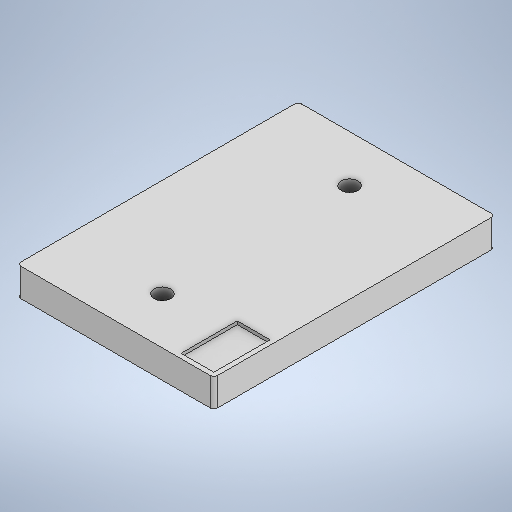
# Autodesk Inventor part: Podstawa
Saved by Autodesk Inventor 2025 (Build 290162000, 162)
## iProperties
Created: 2024-04-05
Part Number: Podstawa
Material: Generic
Document SubType Name: Modeling
Designer: Wojtek
Density: 1 g/cm^3
Appearance: Default
Author: Wojtek
Autodesk Inventor part; units mm, degrees
ref_plane "YZ Plane" through (0, 0, 0) normal (1, 0, 0) x (0, 1, 0)
ref_plane "XZ Plane" through (0, 0, 0) normal (0, 1, 0) x (-1, 0, 0)
ref_plane "XY Plane" through (0, 0, 0) normal (0, 0, 1) x (1, 0, 0)
sketch "Sketch1" plane through (0, 0, 0) normal (0, 1, 0) x (-1, 0, 0)
  line L0 (105, -150) -> (-105, -150)
  line L1 (-105, -150) -> (-105, 150)
  line L2 (-105, 150) -> (105, 150)
  line L3 (105, 150) -> (105, -150)
  line L4 (105, -150) -> (-105, 150) construction
  line L5 (-105, -150) -> (105, 150) construction
  point P0 (0, 0)
  dimension "d0" = 210
  dimension "d1" = 300
  constraints: 12 end point, 2 midpoint, 2 parallel, 1 horizontal, 1 perpendicular
  measures "d0" distance of L1.end L2.end
  measures "d1" distance of L0.end L1.end
extrude "Extrusion1" add sketch "Sketch1" along normal blind 30
sketch "Sketch2" plane through (0, 30, 0) normal (0, 1, 0) x (1, 0, 0)
  circle A0 centre (0, 100) radius 9
  circle A1 centre (0, -100) radius 9
  point P0 (0, 0)
  dimension "d4" = 18
  dimension "d5" = 18
  dimension "d6" = 100
  dimension "d7" = 100
  constraints: 2 centre point, 2 vertical alignment
  measures "d4" diameter of A0
  measures "d5" diameter of A1
  measures "d6" distance of point (0, 0) A0.centre
  measures "d7" distance of point (0, 0) A1.centre
hole "Hole1" at (0, 30, -100) at (0, 30, 100) direction (0, -1, 0) diameter 0.1 end through all counterbore diameter 18 counterbore depth 24
sketch "Sketch3" plane through (0, 30, 0) normal (0, 1, 0) x (1, 0, 0)
  line L0 (65, -145) -> (100, -145)
  line L1 (100, -145) -> (100, -85)
  line L2 (100, -85) -> (65, -85)
  line L3 (65, -85) -> (65, -145)
  line L4 (-105, -150) -> (105, -150) projected
  line L5 (105, -150) -> (105, 150) projected
  point P0 (0, 0)
  dimension "d15" = 35
  dimension "d16" = 60
  dimension "d17" = 5
  dimension "d19" = 5
  constraints: 8 end point, 2 parallel, 1 horizontal, 1 perpendicular
  measures "d15" distance of L2.end L1.end
  measures "d16" distance of L1.end L0.end
  measures "d17" distance between parallel lines of L4 L0
  measures "d19" distance between parallel lines of L5 L1
extrude "Extrusion2" cut sketch "Sketch3" against normal blind 3.5
fillet "Fillet1" radius 4 4 edges at (105, 15, 150) (-105, 15, 150) (105, 15, -150) (-105, 15, -150)
body "Solid1"
